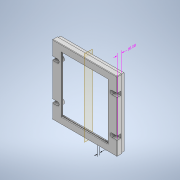
# Autodesk Inventor part: Part_B2
Saved by Autodesk Inventor 2022.6 (Build 266554010, 554A)
## iProperties
Created: 2025-05-15
Part Number: Part_B2
Material: Generic
Document SubType Name: Modeling
Designer: khinm
Density: 1 g/cm^3
Appearance: Default
Author: khinm
Autodesk Inventor part; units mm, degrees
ref_plane "XZ Plane" through (0, 0, 0) normal (0, 1, 0) x (-1, 0, 0)
ref_plane "XY Plane" through (0, 0, 0) normal (0, 0, 1) x (1, 0, 0)
sketch "Sketch1" plane through (0, 0, 0) normal (0, 0, 1) x (1, 0, 0)
  line L0 (-70, 75) -> (70, 75)
  line L1 (70, 75) -> (70, -75)
  line L2 (70, -75) -> (-70, -75)
  line L3 (-70, -75) -> (-70, 75)
  point P0 (0, 0)
  point P1 (-70, 0)
  point P2 (0, 75)
  dimension "d0" = 140
  dimension "d1" = 150
  constraints: 8 end point, 2 midpoint, 2 parallel, 1 horizontal, 1 horizontal alignment, 1 perpendicular, 1 vertical alignment
  measures "d0" distance of L0.start L0.end
  measures "d1" distance of L0.end L1.end
extrude "Extrusion1" add sketch "Sketch1" along normal mid plane 10
fillet "Fillet1" radius 1 4 edges at (70, 75, 0) (70, -75, 0) (-70, 75, 0) (-70, -75, 0)
sketch "Sketch2" plane through (0, 0, -5) normal (0, 0, -1) x (-1, 0, 0)
  line L0 (-65, 70) -> (65, 70)
  line L1 (65, 70) -> (65, -70)
  line L2 (65, -70) -> (-65, -70)
  line L3 (-65, -70) -> (-65, 70)
  point P0 (0, 0)
  point P1 (0, 70)
  point P2 (-65, 0)
  dimension "d5" = 130
  dimension "d6" = 140
  constraints: 8 end point, 2 midpoint, 2 parallel, 1 horizontal, 1 horizontal alignment, 1 perpendicular, 1 vertical alignment
  measures "d5" distance of L0.start L0.end
  measures "d6" distance of L2.end L0.start
extrude "Extrusion2" cut sketch "Sketch2" against normal blind 5
ref_plane "Work Plane1" through (0, 0, 0) normal (1, 0, 0) x (0, 1, 0)
sketch "Sketch3" plane through (0, 0, 0) normal (1, 0, 0) x (0, 1, 0)
  line L0 (70, -5) -> (70, 0) projected
  line L1 (-74, -5) -> (74, -5) projected
  line L2 (75, -5) -> (74, -5) projected
  line L3 (73.49, -5) -> (71.51, -5)
  line L4 (71.51, -5) -> (71.51, -11.5)
  line L5 (71.51, -11.5) -> (73.49, -11.5)
  line L6 (73.49, -11.5) -> (73.49, -5)
  line L7 (75, -5) -> (70, -5)
  point P0 (0, 0)
  point P1 (71.51, -8.25)
  point P2 (72.5, -5)
  point P3 (72.5, -5)
  dimension "d10" = 6.5
  dimension "d12" = 1.98
  dimension "d13" = 0
  constraints: 10 end point, 3 midpoint, 2 parallel, 1 coincident, 1 collinear, 1 horizontal, 1 perpendicular
  measures "d10" distance of L5.end L3.start
  measures "d12" distance of L5.end L4.end
  measures "d13" distance between parallel lines of L1 L3
sketch3d "3D Sketch1"
  line L0 (65, 70, -5) -> (65, -70, -5)
  line L1 (65, -70, -5) -> (-65, -70, -5)
  line L2 (-65, -70, -5) -> (-65, 70, -5)
  line L3 (-65, 70, -5) -> (65, 70, -5)
sweep "Sweep1" add profiles "Sketch3" path "3D Sketch1"
sketch "Sketch4" plane through (0, 0, 0) normal (0, 0, -1) x (-1, 0, 0)
  arc A0 (-59, 34.5) -> (-59, 45.5) centre (-59, 40) ccw
  line L0 (-65, -70) -> (-65, 70) projected
  line L1 (-65, 70) -> (65, 70) projected
  line L2 (-59, 34.5) -> (-65, 34.5)
  line L3 (-59, 45.5) -> (-65, 45.5)
  line L4 (-65, -70) -> (-65, 70) projected
  line L5 (-65, 34.5) -> (-65, 45.5)
  arc A1 (-59, -45.5) -> (-59, -34.5) centre (-59, -40) ccw
  line L6 (65, -70) -> (-65, -70) projected
  line L7 (-59, -45.5) -> (-65, -45.5)
  line L8 (-59, -34.5) -> (-65, -34.5)
  line L9 (-65, -45.5) -> (-65, -34.5)
  point P0 (0, 0)
  dimension "d16" = 6
  dimension "d17" = 11
  dimension "d18" = 30
  dimension "d19" = 30
  dimension "d20" = 6
  dimension "d21" = 11
  constraints: 12 end point, 4 point on circle, 4 point on line, 4 tangent, 3 perpendicular, 2 centre point, 2 collinear, 1 horizontal
  measures "d16" distance from line of L0 A0.centre
  measures "d17" diameter of A0
  measures "d18" distance from line of L1 A0.centre
  measures "d19" distance from line of L6 A1.centre
  measures "d20" distance from line of L0 A1.centre
  measures "d21" diameter of A1
extrude "Extrusion3" add sketch "Sketch4" along normal up to surface (5 mm away)
sketch "Sketch7" plane through (0, 0, 5) normal (0, 0, 1) x (1, 0, 0)
  arc A0 (59, 45.5) -> (59, 34.5) centre (59, 40) ccw projected
  arc A1 (59, 44) -> (59, 36) centre (59, 40) ccw
  line L0 (70, -74) -> (70, 74) projected
  line L1 (59, 36) -> (70, 36)
  line L2 (70, 74) -> (70, -74) projected
  line L3 (59, 44) -> (70, 44)
  line L4 (70, 36) -> (70, 44)
  arc A2 (59, -34.5) -> (59, -45.5) centre (59, -40) ccw projected
  arc A3 (59, -36) -> (59, -44) centre (59, -40) ccw
  line L5 (59, -44) -> (70, -44)
  line L6 (59, -36) -> (70, -36)
  line L7 (70, -44) -> (70, -36)
  point P0 (0, 0)
  dimension "d37" = 8
  dimension "d40" = 8
  constraints: 12 end point, 4 perpendicular, 4 point on circle, 4 point on line, 4 tangent, 2 centre point, 2 coincident, 1 collinear, 1 parallel
  measures "d37" diameter of A1
  measures "d40" diameter of A3
extrude "Extrusion5" cut sketch "Sketch7" against normal blind 8
mirror "Mirror1" about plane through (0, 0, 0) normal (1, 0, 0) of "Extrusion5", "Extrusion3"
sketch "Sketch8" plane through (0, 0, -5) normal (0, 0, -1) x (-1, 0, 0)
  arc A0 (-59, 34.5) -> (-59, 45.5) centre (-59, 40) ccw projected
  arc A1 (59, 44) -> (59, 36) centre (59, 40) ccw projected
  arc A2 (-59, -44) -> (-59, -36) centre (-59, -40) ccw projected
  arc A3 (59, -34.5) -> (59, -45.5) centre (59, -40) ccw projected
  point P0 (0, 0)
  constraints: 4 coincident
hole "Hole1" at (59, 40, -5) at (-59, 40, -5) at (59, -40, -5) at (-59, -40, -5) direction (0, 0, 1) diameter 2.013 depth 2
sketch "Sketch9" plane through (0, 0, 5) normal (0, 0, 1) x (1, 0, 0)
  line L0 (-50, 60) -> (50, 60)
  line L1 (50, 60) -> (50, -60)
  line L2 (50, -60) -> (-50, -60)
  line L3 (-50, -60) -> (-50, 60)
  line L4 (-70, 36) -> (-70, -36) projected
  point P0 (0, 0)
  point P1 (0, 60)
  point P2 (-50, 0)
  point P3 (-70, 0)
  dimension "d48" = 100
  dimension "d49" = 120
  constraints: 8 end point, 3 midpoint, 2 parallel, 1 horizontal, 1 horizontal alignment, 1 perpendicular, 1 vertical alignment
  measures "d48" distance of L0.start L0.end
  measures "d49" distance between parallel lines of L2 L0
extrude "Extrusion6" cut sketch "Sketch9" against normal up to surface (5 mm away)
sketch "Sketch10" plane through (0, 0, 0) normal (0, 0, -1) x (-1, 0, 0)
  line L0 (-52.5, 62.5) -> (52.5, 62.5)
  line L1 (52.5, 62.5) -> (52.5, -62.5)
  line L2 (52.5, -62.5) -> (-52.5, -62.5)
  line L3 (-52.5, -62.5) -> (-52.5, 62.5)
  point P0 (0, 0)
  point P1 (0, 62.5)
  point P2 (-52.5, 0)
  dimension "d52" = 105
  dimension "d53" = 125
  constraints: 8 end point, 2 midpoint, 2 parallel, 1 horizontal, 1 horizontal alignment, 1 perpendicular, 1 vertical alignment
  measures "d52" distance of L0.start L0.end
  measures "d53" distance of L0.end L1.end
extrude "Extrusion7" cut sketch "Sketch10" against normal blind 3
chamfer "Chamfer1" distance 1 angle 45 4 edges at (-50, 0, 5) (0, 60, 5) (50, 0, 5) (0, -60, 5)
fillet "Fillet2" radius 1 12 edges at (-69.7071, 74.7071, 5) (-70, 59, 5) (69.7071, 74.7071, 5) (70, 59, 5) (0, 75, 5) (70, 0, 5) (69.7071, -74.7071, 5) (0, -75, 5) (-69.7071, -74.7071, 5) (-70, -59, 5) (70, -59, 5) (-70, 0, 5)
body "Solid1"
